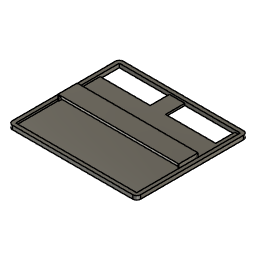
Center Side Up Cover 2x1 v4 (Autodesk Fusion 360 design; units mm, degrees)
Autodesk Fusion 360 part; units mm, degrees
sketch "Schizzo1" plane through (0, 0, 0) normal (0, 0, 1) x (1, 0, 0)
  line L0 (29.4832, 68.3919) -> (96.1832, 68.3919) construction
  line L1 (96.1832, 68.3919) -> (96.1832, 10.6919) construction
  line L2 (96.1832, 10.6919) -> (29.4832, 10.6919) construction
  line L3 (29.4832, 10.6919) -> (29.4832, 68.3919) construction
  line L4 (96.0832, 10.7919) -> (29.5832, 10.7919)
  line L5 (29.5832, 10.7919) -> (29.5832, 68.2919)
  line L6 (29.5832, 68.2919) -> (96.0832, 68.2919)
  line L7 (96.0832, 68.2919) -> (96.0832, 10.7919)
  line L8 (94.1832, 12.6919) -> (31.4832, 12.6919)
  line L9 (31.4832, 12.6919) -> (31.4832, 66.3919)
  line L10 (31.4832, 66.3919) -> (94.1832, 66.3919)
  line L11 (94.1832, 66.3919) -> (94.1832, 12.6919)
  line L12 (31.4832, 66.3919) -> (57.4832, 66.3919)
  line L13 (57.4832, 66.3919) -> (57.4832, 56.3919)
  line L14 (57.4832, 56.3919) -> (31.4832, 56.3919)
  line L15 (31.4832, 56.3919) -> (31.4832, 66.3919)
  line L16 (65.4832, 66.3919) -> (91.4832, 66.3919)
  line L17 (91.4832, 56.3919) -> (65.4832, 56.3919)
  line L18 (91.4832, 66.3919) -> (91.4832, 56.3919)
  line L19 (65.4832, 56.3919) -> (65.4832, 66.3919)
  line L20 (29.4832, 39.5419) -> (96.1832, 39.5419) construction
  line L21 (31.4832, 44.5419) -> (94.1832, 44.5419)
  line L22 (31.4832, 34.5419) -> (94.1832, 34.5419)
  line L23 (62.8332, 68.3919) -> (62.8332, 10.7919) construction
  dimension "d1" = 66.7
  dimension "d2" = 57.7
  dimension "d3" = 0.1
  dimension "d4" = 2
  dimension "d5" = 26
  dimension "d6" = 10
  dimension "d9" = 34
  dimension "d10" = 0
  dimension "d16" = 10
  constraint horizontal L0
  constraint vertical L1
  constraint horizontal L2
  constraint vertical L3
  constraint horizontal L12
  constraint vertical L13
  constraint horizontal L14
  constraint vertical L15
  constraint midpoint L3 L20.start
  constraint midpoint L1 L20.end
  constraint coincident L9 L21.start
  constraint coincident L11 L21.end
  constraint perpendicular L11 L21
  constraint symmetric L20 L21.start L22.start
  constraint symmetric L20 L21.end L22.end
  constraint midpoint L0 L23.start
  constraint midpoint L4 L23.end
  measures "d1" distance of L0.start L0.end
  measures "d2" distance of L0.start L2.end
  measures "d5" distance of L9.end L12.end
  measures "d6" distance of L9.end L14.end
  measures "d16" distance of L21 L22
extrude "Estrusione1" add sketch "Schizzo1" along normal blind 1 contours L8 L9 L11 L22 | L9 L11 L21 L22 | L9 L10 L11 L13 L14 L17 L18 L19 L21
extrude "Estrusione2" add sketch "Schizzo1" along normal blind 2
fillet "Raccordo1" radius 2 4 edges at (29.5832, 10.7919, 1) (96.0832, 10.7919, 1) (96.0832, 68.2919, 1) (29.5832, 68.2919, 1)
extrude "Estrusione3" add sketch "Schizzo1" along normal blind 4 contours L9 L11 L21 L22
ref_plane "Piano di lavoro1" through (62.8332, 39.5919, 0) normal (-1, 0, 0) x (0, -1, 0)
sketch "Schizzo2" plane through (62.8332, 0, 0) normal (-1, 0, 0) x (0, -1, 0)
  line L0 (-34.5419, 1) -> (-44.5419, 1) construction
  line L1 (-34.5419, 1) -> (-34.5419, 4)
  line L2 (-34.5419, 4) -> (-36.274, 1)
  line L3 (-36.274, 1) -> (-34.5419, 1)
  line L4 (-39.5419, 1) -> (-39.5419, 4) construction
  line L5 (-44.5419, 4) -> (-34.5419, 4) construction
  line L6 (-44.5419, 4) -> (-42.8099, 1)
  line L7 (-42.8099, 1) -> (-44.5419, 1)
  line L8 (-44.5419, 1) -> (-44.5419, 4)
  point P0 (-34.5419, 1)
  point P1 (-44.5419, 1)
  dimension "d20" = 30
  constraint horizontal L0
  constraint coincident P0 L0.start
  constraint coincident P1 L0.end
  constraint perpendicular L0 L1
  constraint coincident L0 L2.end
  constraint perpendicular L1 L3
  constraint midpoint L0 L4.start
  constraint perpendicular L0 L4
  constraint coincident L4.end L5
  constraint symmetric P0 L4 L0.end
  constraint symmetric L1.end L4 L5.start
  constraint symmetric L2.end L4 L6.end
  constraint symmetric P0 L4 P1
  measures "d20" angle of L1 L2
extrude "Estrusione4" cut sketch "Schizzo2" along normal mid plane 62
